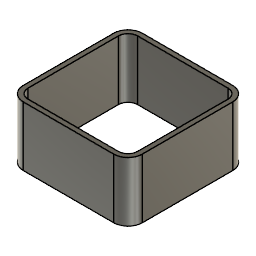
▢-200×200×8.0 (Autodesk Fusion 360 design; units mm, degrees)
Autodesk Fusion 360 part; units mm, degrees
sketch "スケッチ1" plane through (0, 0, 0) normal (0, 0, 1) x (1, 0, 0)
  line L0 (942.8497, -699.0501) -> (942.8497, -547.0501)
  line L1 (934.8497, -699.0501) -> (934.8497, -547.0501)
  line L2 (742.8497, -547.0501) -> (742.8497, -699.0501)
  line L3 (750.8497, -547.0501) -> (750.8497, -699.0501)
  line L4 (766.8497, -723.0501) -> (918.8497, -723.0501)
  line L5 (766.8497, -715.0501) -> (918.8497, -715.0501)
  arc A0 (742.8497, -699.0501) -> (766.8497, -723.0501) centre (766.8497, -699.0501) ccw
  arc A1 (750.8497, -699.0501) -> (766.8497, -715.0501) centre (766.8497, -699.0501) ccw
  arc A2 (918.8497, -723.0501) -> (942.8497, -699.0501) centre (918.8497, -699.0501) ccw
  arc A3 (918.8497, -715.0501) -> (934.8497, -699.0501) centre (918.8497, -699.0501) ccw
  line L6 (918.8497, -523.0501) -> (766.8497, -523.0501)
  line L7 (918.8497, -531.0501) -> (766.8497, -531.0501)
  arc A4 (766.8497, -523.0501) -> (742.8497, -547.0501) centre (766.8497, -547.0501) ccw
  arc A5 (766.8497, -531.0501) -> (750.8497, -547.0501) centre (766.8497, -547.0501) ccw
  arc A6 (942.8497, -547.0501) -> (918.8497, -523.0501) centre (918.8497, -547.0501) ccw
  arc A7 (934.8497, -547.0501) -> (918.8497, -531.0501) centre (918.8497, -547.0501) ccw
  point P0 (842.8497, -623.0501)
extrude "押し出し1" add sketch "スケッチ1" along normal blind 100
